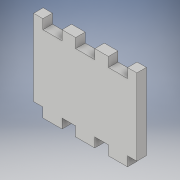
# Autodesk Inventor part: front-flat
Saved by Autodesk Inventor 2018 (Build 220112000, 112)
## iProperties
Created: 2018-03-29
Part Number: front-flat
Material: Generic
Document SubType Name: Modeling
Designer: guita
Density: 1 g/cm^3
Appearance: Default
Author: guita
Autodesk Inventor part; units mm, degrees
ref_plane "YZ Plane" through (0, 0, 0) normal (1, 0, 0) x (0, 1, 0)
ref_plane "XZ Plane" through (0, 0, 0) normal (0, 1, 0) x (-1, 0, 0)
ref_plane "XY Plane" through (0, 0, 0) normal (0, 0, 1) x (1, 0, 0)
sketch "Sketch1" plane through (0, 0, 0) normal (0, 0, 1) x (1, 0, 0)
  line L0 (68.58, 6.35) -> (68.58, 57.15)
  line L1 (68.58, 57.15) -> (0, 57.15)
  line L2 (0, 57.15) -> (0, 6.35)
  line L3 (40.64, 6.35) -> (40.64, 0)
  line L4 (27.94, 6.35) -> (27.94, 0)
  line L5 (27.94, 0) -> (40.64, 0)
  line L6 (27.94, 6.35) -> (18.8722, 6.35)
  line L7 (18.8722, 6.35) -> (18.8722, 0)
  line L8 (18.8722, 0) -> (6.1722, 0)
  line L9 (6.1722, 0) -> (6.1722, 6.35)
  line L10 (40.64, 6.35) -> (49.7078, 6.35)
  line L11 (49.7078, 6.35) -> (49.7078, 0)
  line L12 (49.7078, 0) -> (62.4078, 0)
  line L13 (62.4078, 0) -> (62.4078, 6.35)
  line L14 (6.1722, 0) -> (18.8722, 0)
  line L15 (27.94, 0) -> (40.64, 0)
  line L16 (49.7078, 0) -> (62.4078, 0)
  line L17 (27.94, 6.35) -> (18.8722, 6.35)
  line L18 (6.1722, 6.35) -> (0, 6.35)
  line L19 (40.64, 6.35) -> (49.7078, 6.35)
  line L20 (62.4078, 6.35) -> (68.58, 6.35)
  point P0 (0, 0)
  dimension "d0" = 68.58
  dimension "d1" = 50.8
  constraints: 42 end point, 23 perpendicular, 4 parallel, 3 collinear, 3 horizontal
  measures "d0" distance of L1.end L0.end
  measures "d1" distance of L0.end L0.start
extrude "Extrusion1" add sketch "Sketch1" against normal blind 6.35
sketch "Sketch2" plane through (0, 0, 0) normal (0, 0, 1) x (1, 0, 0)
  line L0 (0, 6.35) -> (6.1722, 6.35) projected
  line L1 (6.1722, 50.8) -> (6.1722, 57.15)
  line L2 (0, 57.15) -> (68.58, 57.15) projected
  line L3 (49.7078, 6.35) -> (40.64, 6.35) projected
  line L4 (40.64, 50.8) -> (40.64, 57.15)
  line L5 (18.8722, 0) -> (18.8722, 6.35) projected
  line L6 (18.8722, 50.8) -> (18.8722, 57.15)
  line L7 (27.94, 0) -> (27.94, 6.35) projected
  line L8 (27.94, 50.8) -> (27.94, 57.15)
  line L9 (49.7078, 50.8) -> (49.7078, 57.15)
  line L10 (68.58, 6.35) -> (62.4078, 6.35) projected
  line L11 (62.4078, 50.8) -> (62.4078, 57.15)
  line L12 (0, 57.15) -> (0, 50.8)
  line L13 (68.58, 57.15) -> (68.58, 6.35) projected
  line L14 (49.7078, 50.8) -> (62.4078, 50.8)
  line L15 (6.1722, 50.8) -> (18.8722, 50.8)
  line L16 (27.94, 50.8) -> (40.64, 50.8)
  line L17 (27.94, 57.15) -> (40.64, 57.15)
  point P0 (0, 0)
  constraints: 22 end point, 7 perpendicular, 5 point on line, 2 vertical, 1 collinear, 1 parallel
extrude "Extrusion2" cut sketch "Sketch2" against normal blind 6.35
sketch "Sketch3" plane through (0, 0, -6.35) normal (0, 0, -1) x (-1, 0, 0)
  line L0 (-63.699, 7.8373) -> (-3.501, 7.8373)
  line L1 (-3.501, 7.8373) -> (-3.501, 47.2073)
  line L2 (-3.501, 47.2073) -> (-63.699, 47.2073)
  line L3 (-63.699, 47.2073) -> (-63.699, 7.8373)
  point P0 (0, 0)
  dimension "d15" = 60.198
  dimension "d16" = 39.37
  constraints: 8 end point, 2 horizontal, 1 perpendicular, 1 vertical
  measures "d15" distance of L0.start L0.end
  measures "d16" distance of L0.end L1.end
extrude "Extrusion3" cut sketch "Sketch3" against normal blind 3.81
body "Solid1"
